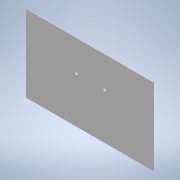
# Autodesk Inventor part: CONTROL_BREEDTE
Saved by Autodesk Inventor 2020 (Build 240168000, 168)
## iProperties
Created: 2020-06-03
Part Number: CONTROL_BREEDTE
Material: Generic
Document SubType Name: Sheet Metal
Designer: Gebruiker
Density: 1 g/cm^3
Sheet Metal Rule: Default_mm
Appearance: Default
Author: Gebruiker
Autodesk Inventor part; units mm, degrees
ref_plane "YZ Plane" through (0, 0, 0) normal (1, 0, 0) x (0, 1, 0)
ref_plane "XZ Plane" through (0, 0, 0) normal (0, 1, 0) x (-1, 0, 0)
ref_plane "XY Plane" through (0, 0, 0) normal (0, 0, 1) x (1, 0, 0)
sketch "Sketch1" plane through (0, 0, 0) normal (0, 0, 1) x (1, 0, 0)
  line L0 (-125, 75) -> (125, 75)
  line L1 (125, 75) -> (125, -75)
  line L2 (125, -75) -> (-125, -75)
  line L3 (-125, -75) -> (-125, 75)
  line L4 (-125, 75) -> (125, -75) construction
  line L5 (125, 75) -> (-125, -75) construction
  point P0 (0, 0)
  dimension "d0" = 250
  dimension "d1" = 150
  measures "d0" distance of L1.end L2.end
  measures "d1" distance of L0.end L1.end
extrude "Plate1" add sketch "Sketch1" along normal blind 0.5
sketch "Sketch3" plane through (0, 0, 0.5) normal (0, 0, 1) x (1, 0, 0)
  circle A0 centre (-26.2041, 14.6677) radius 2.25 projected
  circle A1 centre (28.7959, 14.6677) radius 2.25 projected
  point P0 (0, 0)
extrude "Cut1" cut sketch "Sketch3" against normal blind 0.5
equation "\"d13\" = Thickness"
equation "\"d2\" = Thickness"
equation "\"BendRadius\" = Thickness"
equation "\"BendReliefWidth\" = Thickness"
equation "\"BendReliefDepth\" = 0.5 * Thickness"
equation "\"CornerReliefSize\" = 4 * Thickness"
equation "\"MinimumRemnant\" = 2 * Thickness"
equation "\"TransitionRadius\" = BendRadius"
equation "\"JacobiRadiusSize\" = BendRadius"
equation "\"GapSize\" = Thickness"
equation "\"Thickness\" = 0.5"
body "Solid1"
